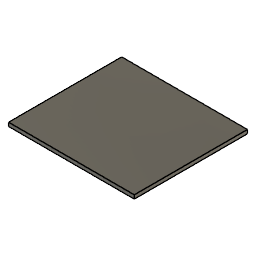
Assemble (Autodesk Fusion 360 archive; units mm, degrees)
design "PCB"
part number: 2026-03-31-20-07-59-001
Autodesk Fusion 360 part; units mm, degrees
sketch "Boceto1" plane through (0, 0, 0) normal (0, 0, 1) x (1, 0, 0)
  line L0 (50, -45) -> (-50, -45)
  line L1 (-50, -45) -> (-50, 45)
  line L2 (-50, 45) -> (50, 45)
  line L3 (50, 45) -> (50, -45)
  line L4 (50, -45) -> (-50, 45) construction
  line L5 (-50, -45) -> (50, 45) construction
  dimension "d1" = 100
  dimension "d2" = 90
  constraint horizontal L0
  constraint perpendicular L0 L1
  constraint parallel L0 L2
  constraint parallel L1 L3
  constraint coincident L4 origin
  constraint coincident L5 origin
  measures "d1" distance of L1.end L2.end
  measures "d2" distance of L0.end L1.end
extrude "Extruir1" add sketch "Boceto1" along normal blind 3

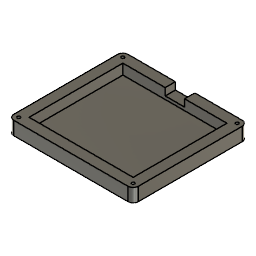
design "Bottom"
part number: 2026-03-31-19-47-08-928
Autodesk Fusion 360 part; units mm, degrees
sketch "Boceto1" plane through (0, 0, 0) normal (0, 0, 1) x (1, 0, 0)
  line L0 (50.5, -45.5) -> (-50.5, -45.5)
  line L1 (-50.5, -45.5) -> (-50.5, 45.5)
  line L2 (-50.5, 45.5) -> (50.5, 45.5)
  line L3 (50.5, 45.5) -> (50.5, -45.5)
  line L4 (50.5, -45.5) -> (-50.5, 45.5) construction
  line L5 (-50.5, -45.5) -> (50.5, 45.5) construction
  line L6 (60.5, -55.5) -> (-60.5, -55.5)
  line L7 (-60.5, -55.5) -> (-60.5, 55.5)
  line L8 (-60.5, 55.5) -> (60.5, 55.5)
  line L9 (60.5, 55.5) -> (60.5, -55.5)
  line L10 (60.5, -55.5) -> (-60.5, 55.5) construction
  line L11 (-60.5, -55.5) -> (60.5, 55.5) construction
  circle A0 centre (55.5, 50.5) radius 1.45
  circle A1 centre (55.5, -50.5) radius 1.45
  circle A2 centre (-55.5, -50.5) radius 1.45
  circle A3 centre (-55.5, 50.5) radius 1.45
  dimension "d1" = 101
  dimension "d2" = 91
  dimension "d3" = 121
  dimension "d4" = 111
  dimension "d6" = 2.9
  dimension "d10" = 2.9
  dimension "d11" = 2.9
  dimension "d12" = 2.9
  constraint horizontal L0
  constraint perpendicular L0 L1
  constraint parallel L0 L2
  constraint parallel L1 L3
  constraint coincident L4 origin
  constraint coincident L5 origin
  constraint horizontal L6
  constraint perpendicular L6 L7
  constraint parallel L6 L8
  constraint parallel L7 L9
  constraint coincident L10 origin
  constraint coincident L11 origin
  measures "d1" distance of L1.end L2.end
  measures "d2" distance of L0.end L1.end
  measures "d3" distance of L7.end L8.end
  measures "d4" distance of L6.end L7.end
  measures "d6" diameter of A0
  measures "d10" diameter of A1
  measures "d11" diameter of A2
  measures "d12" diameter of A3
extrude "Extruir1" add sketch "Boceto1" along normal blind 3 contours L0 L1 L2 L3
extrude "Extruir2" add sketch "Boceto1" along normal blind 13
sketch "Boceto2" plane through (0, 0, 13) normal (0, 0, 1) x (-1, 0, 0)
  circle A0 centre (55.5, 50.5) radius 1.45
  line L0 (50.5, -45.5) -> (-50.5, -45.5)
  line L1 (-50.5, -45.5) -> (-50.5, 45.5)
  line L2 (-50.5, 45.5) -> (50.5, 45.5)
  line L3 (50.5, 45.5) -> (50.5, -45.5)
  circle A1 centre (55.5, -50.5) radius 1.45
  circle A2 centre (-55.5, -50.5) radius 1.45
  circle A3 centre (-55.5, 50.5) radius 1.45
  line L4 (-60.5, -55.5) -> (60.5, -55.5)
  line L5 (60.5, -55.5) -> (60.5, 55.5)
  line L6 (60.5, 55.5) -> (-60.5, 55.5)
  line L7 (-60.5, 55.5) -> (-60.5, -55.5)
  line L8 (50.5, -45.5) -> (9.404, -45.5)
  line L9 (9.404, -45.5) -> (9.404, -55.5)
  line L10 (9.404, -55.5) -> (50.5, -55.5)
  line L11 (50.5, -55.5) -> (50.5, -45.5)
  line L12 (9.404, -55.5) -> (-9.396, -55.5)
  line L13 (-9.396, -55.5) -> (-9.396, -45.5)
  line L14 (-9.396, -45.5) -> (9.404, -45.5)
  line L15 (9.404, -45.5) -> (9.404, -55.5)
  line L16 (-9.396, -55.5) -> (-50.5, -55.5)
  line L17 (-50.5, -55.5) -> (-50.5, -45.5)
  line L18 (-50.5, -45.5) -> (-9.396, -45.5)
  line L19 (-9.396, -45.5) -> (-9.396, -55.5)
  dimension "d17" = 41.096
  dimension "d18" = 18.8
  constraint horizontal L8
  constraint vertical L9
  constraint horizontal L10
  constraint vertical L11
  constraint coincident L0.start L3.end
  constraint horizontal L12
  constraint vertical L13
  constraint horizontal L14
  constraint vertical L15
  constraint horizontal L16
  constraint vertical L17
  constraint horizontal L18
  constraint vertical L19
  constraint coincident L0.end L1.start
  measures "d17" distance of L0.start L8.end
  measures "d18" distance of L9.end L12.end
extrude "Extruir3" cut sketch "Boceto2" against normal blind 7 contours L0 L4 L9 L12 L13 L14 L15 L19
fillet "Empalme1" radius 5 4 edges at (60.5, 55.5, 6.5) (60.5, -55.5, 6.5) (-60.5, -55.5, 6.5) (-60.5, 55.5, 6.5)
sketch "Boceto3" plane through (0, 0, 0) normal (0, 0, 1) x (1, 0, 0)
  line L0 (29.725, -4.2847) -> (-29.5911, -4.2847) construction
  line L1 (-29.5911, -4.2847) -> (-29.5911, 6.6948) construction
  line L2 (-29.5911, 6.6948) -> (29.725, 6.6948) construction
  line L3 (29.725, 6.6948) -> (29.725, -4.2847) construction
  dimension "d23" = 15
  text T0 "NeowPad" font "Arial" height 15 bold align centre middle in box 59.3161 x 10.9795 at (29.725, -4.2847) x (-1, 0) y (0, 1) spacing 1 kerned
extrude "Extruir4" cut sketch "Boceto3" along normal blind 1 text T0
equation "d1 = 100 mm + 1 mm"
equation "d2 = 90 mm + 1 mm"
equation "d3 = 100 mm + 1 mm + 20 mm"
equation "d4 = 90 mm + 1 mm + 20 mm"
equation "d18 = 17.8 mm + 1 mm"
equation "d24 = 'NeowPad'"

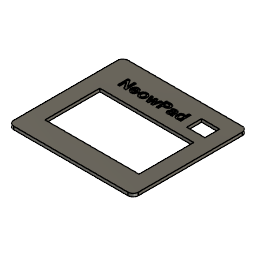
design "Top"
part number: 2026-03-31-19-46-04-300
Autodesk Fusion 360 part; units mm, degrees
sketch "Boceto1" plane through (0, 0, 0) normal (0, 0, 1) x (1, 0, 0)
  line L0 (60.5, -55.5) -> (-60.5, -55.5)
  line L1 (-60.5, -55.5) -> (-60.5, 55.5)
  line L2 (-60.5, 55.5) -> (60.5, 55.5)
  line L3 (60.5, 55.5) -> (60.5, -55.5)
  line L4 (60.5, -55.5) -> (-60.5, 55.5) construction
  line L5 (-60.5, -55.5) -> (60.5, 55.5) construction
  line L6 (50.5, -45.5) -> (-50.5, 45.5) construction
  line L7 (-50.5, -45.5) -> (50.5, 45.5) construction
  line L8 (-50.5, -45.5) -> (-45.585, -45.5)
  line L9 (-45.585, -34.875) -> (-50.5, -34.875)
  line L10 (-50.5, -34.875) -> (-50.5, -45.5)
  line L11 (50.5, -45.5) -> (45.585, -45.5)
  line L12 (45.585, -34.875) -> (50.5, -34.875)
  line L13 (50.5, -34.875) -> (50.5, -45.5)
  line L14 (-45.585, -34.875) -> (45.585, -34.875)
  line L15 (45.585, -34.875) -> (45.585, 18.195)
  line L16 (45.585, 18.195) -> (-45.585, 18.195)
  line L17 (-45.585, 18.195) -> (-45.585, -34.875)
  line L18 (50.5, 45.5) -> (46.85, 45.5)
  line L19 (46.85, 41.98) -> (50.5, 41.98)
  line L20 (50.5, 41.98) -> (50.5, 45.5)
  line L21 (46.85, 41.98) -> (29.35, 41.98)
  line L22 (29.35, 41.98) -> (29.35, 27.78)
  line L23 (29.35, 27.78) -> (46.85, 27.78)
  line L24 (46.85, 27.78) -> (46.85, 41.98)
  dimension "d1" = 121
  dimension "d2" = 111
  dimension "d3" = 101
  dimension "d4" = 91
  dimension "d5" = 4.915
  dimension "d6" = 10.625
  dimension "d7" = 4.915
  dimension "d8" = 10.625
  dimension "d10" = 53.07
  dimension "d11" = 3.65
  dimension "d12" = 3.52
  dimension "d13" = 17.5
  dimension "d14" = 14.2
  constraint horizontal L0
  constraint perpendicular L0 L1
  constraint parallel L0 L2
  constraint parallel L1 L3
  constraint coincident L4 origin
  constraint coincident L5 origin
  constraint coincident L6 origin
  constraint coincident L7 origin
  constraint horizontal L8
  constraint horizontal L9
  constraint vertical L10
  constraint horizontal L11
  constraint horizontal L12
  constraint vertical L13
  constraint horizontal L14
  constraint vertical L15
  constraint horizontal L16
  constraint vertical L17
  constraint horizontal L18
  constraint horizontal L19
  constraint vertical L20
  constraint horizontal L21
  constraint vertical L22
  constraint horizontal L23
  constraint vertical L24
  measures "d1" distance of L1.end L2.end
  measures "d2" distance of L0.end L1.end
  measures "d3" distance of L6.end L7.end
  measures "d4" distance of L7.start L6.end
  measures "d5" distance of L7.start L8.end
  measures "d6" distance of L7.start L9.end
  measures "d7" distance of L6.start L11.end
  measures "d8" distance of L6.start L12.end
  measures "d10" distance of L9.start L16.end
  measures "d11" distance of L7.end L18.end
  measures "d12" distance of L7.end L19.end
  measures "d13" distance of L19.start L21.end
  measures "d14" distance of L19.start L23.end
extrude "Extruir1" add sketch "Boceto1" along normal blind 3
sketch "Boceto2" plane through (0, 0, 3) normal (0, 0, 1) x (-1, 0, 0)
  line L0 (-46.85, -41.98) -> (-46.85, -27.78)
  line L1 (-46.85, -27.78) -> (-29.35, -27.78)
  line L2 (-29.35, -27.78) -> (-29.35, -41.98)
  line L3 (-29.35, -41.98) -> (-46.85, -41.98)
  line L4 (45.585, 34.875) -> (45.585, -18.195)
  line L5 (45.585, -18.195) -> (-45.585, -18.195)
  line L6 (-45.585, -18.195) -> (-45.585, 34.875)
  line L7 (-45.585, 34.875) -> (45.585, 34.875)
  line L8 (-60.5, -55.5) -> (60.5, -55.5)
  line L9 (60.5, -55.5) -> (60.5, 55.5)
  line L10 (60.5, 55.5) -> (-60.5, 55.5)
  line L11 (-60.5, 55.5) -> (-60.5, -55.5)
  line L12 (27.0674, -28.1508) -> (-8.5281, -28.1508) construction
  line L13 (-8.5281, -28.1508) -> (-8.5281, -41.528) construction
  line L14 (-8.5281, -41.528) -> (27.0674, -41.528) construction
  line L15 (27.0674, -41.528) -> (27.0674, -28.1508) construction
  dimension "d17" = 10
  text T0 "NeowPad" font "Arial" height 10 bold align centre middle in box 35.5954 x 13.3772 at (27.0674, -28.1508) x (-1, 0) y (0, -1) spacing 1 kerned
extrude "Extruir2" cut sketch "Boceto2" against normal blind 1 text T0
move_body "Desplazar1" bodies 1 to x (1, 0, 0) y (0, 1, 0) z (0, 0, 1) at (0, 0, -5)
fillet "Empalme1" radius 5 4 edges at (-60.5, -55.5, -3.5) (-60.5, 55.5, -3.5) (60.5, 55.5, -3.5) (60.5, -55.5, -3.5)
equation "d1 = 100 mm + 1 mm + 20 mm"
equation "d2 = 90 mm + 1 mm + 20 mm"
equation "d3 = 100 mm + 1 mm"
equation "d4 = 90 mm + 1 mm"
equation "d11 = 3.15 mm + 0.5 mm"
equation "d12 = 3.02 mm + 0.5 mm"
equation "d18 = 'NeowPad'"
